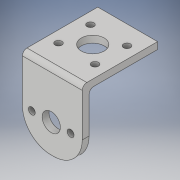
# Autodesk Inventor part: soporte motor
Saved by Autodesk Inventor 2019 (Build 230136000, 136)
## iProperties
Created: 2020-03-05
Part Number: soporte motor
Material: Generic
Document SubType Name: Modeling
Designer: Hugo Albarracin
Density: 1 g/cm^3
Appearance: Default
Author: Hugo Albarracin
Autodesk Inventor part; units mm, degrees
ref_plane "YZ Plane" through (0, 0, 0) normal (1, 0, 0) x (0, 1, 0)
ref_plane "XZ Plane" through (0, 0, 0) normal (0, 1, 0) x (-1, 0, 0)
sketch "Sketch1" plane through (0, 0, 0) normal (1, 0, 0) x (0, 1, 0)
  line L0 (-30.3, 0) -> (0, 0)
  line L1 (0, 0) -> (0, -30)
  line L2 (0, -30) -> (3, -30)
  line L3 (3, -30) -> (3, 3)
  line L4 (3, 3) -> (-30.3, 3)
  line L5 (-30.3, 3) -> (-30.3, 0)
  dimension "d0" = 3
  dimension "d1" = 3
  dimension "d35" = 33.3
  dimension "d36" = 33
  constraints: 12 end point, 5 perpendicular, 1 horizontal
  measures "d0" distance between parallel lines of L3 L1
  measures "d1" distance between parallel lines of L4 L0
  measures "d35" distance between parallel lines of L3 L5
  measures "d36" distance between parallel lines of L2 L4
extrude "Extrusion1" add sketch "Sketch1" along normal mid plane 26.2
fillet "Fillet2" radius 12.5 2 edges at (-13.1, -30.3, 1.5) (13.1, -30.3, 1.5)
ref_plane "Work Plane1" through (13.1, -2, 0) normal (0, 0, -1) x (-1, 0, 0)
sketch "Sketch2" plane through (13.1, -2, 0) normal (0, 0, -1) x (-1, 0, 0)
  circle A0 centre (22.0664, -15.8) radius 1.5
  circle A1 centre (5.0664, -15.8) radius 1.5
  line L0 (22.0664, -15.8) -> (5.0664, -15.8) construction
  line L1 (5.0664, -15.8) -> (0.9327, -15.8) construction
  circle A2 centre (13.5664, -15.8) radius 4
  line L2 (26.2, 2) -> (26.2, -15.8) projected
  line L3 (26.2, -15.8) -> (22.0664, -15.8) construction
  point P0 (13.1, 2)
  dimension "d8" = 3
  dimension "d9" = 3
  dimension "d10" = 17
  dimension "d11" = 8
  constraints: 6 end point, 3 centre point, 1 horizontal, 1 midpoint, 1 point on line
  measures "d8" diameter of A0
  measures "d9" diameter of A1
  measures "d10" distance of L0.end L0.start
  measures "d11" diameter of A2
extrude "Extrusion2" cut sketch "Sketch2" against normal through all
sketch "Sketch6" plane through (-13.1, 3, 3) normal (0, 1, 0) x (1, 0, 0)
  line L0 (26.2, 0) -> (0, 0) projected
  line L1 (26.2, 33) -> (0, 33) projected
  line L2 (13.1, 33) -> (13.1, 0) construction
  circle A0 centre (13.1, 17.7) radius 5
  line L3 (5.1, 24.7) -> (21.1, 24.7) construction
  line L4 (21.1, 24.7) -> (21.1, 10.7) construction
  line L5 (21.1, 10.7) -> (5.1, 10.7) construction
  line L6 (5.1, 10.7) -> (5.1, 24.7) construction
  line L7 (5.1, 24.7) -> (21.1, 10.7) construction
  line L8 (21.1, 24.7) -> (5.1, 10.7) construction
  circle A1 centre (21.1, 10.7) radius 1.5
  circle A2 centre (5.1, 10.7) radius 1.5
  circle A3 centre (5.1, 24.7) radius 1.5
  circle A4 centre (21.1, 24.7) radius 1.5
  point P0 (13.1, 3)
  dimension "d39" = 10
  dimension "d40" = 17.7
  dimension "d41" = 16
  dimension "d42" = 14
  dimension "d43" = 3
  dimension "d44" = 3
  dimension "d45" = 3
  dimension "d46" = 3
  constraints: 14 end point, 5 centre point, 4 coincident, 4 midpoint, 2 parallel, 1 horizontal, 1 perpendicular, 1 point on line
  measures "d39" diameter of A0
  measures "d40" distance from line of L0 A0.centre
  measures "d41" distance of L4.end L5.end
  measures "d42" distance of L3.end L4.end
  measures "d43" diameter of A1
  measures "d44" diameter of A2
  measures "d45" diameter of A3
  measures "d46" diameter of A4
extrude "Extrusion4" cut sketch "Sketch6" against normal up to next
fillet "Fillet3" radius 2 2 edges at (0, 3, 3) (0, 0, 0)
equation "\"d1\" = d0"
body "Solid1"
